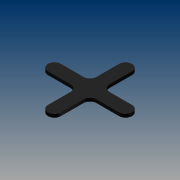
# Autodesk Inventor part: MotorBottom
Saved by Autodesk Inventor 2011 SP1 (Build 150282100, 282)
## iProperties
Created: 2011-07-19
Part Number: MotorBottom
Document SubType Name: Modeling
Designer: Nathan
Density: 1 g/cm^3
Author: Nathan
Autodesk Inventor part; units mm, degrees
ref_plane "YZ Plane" through (0, 0, 0) normal (1, 0, 0) x (0, 1, 0)
ref_plane "XZ Plane" through (0, 0, 0) normal (0, 1, 0) x (-1, 0, 0)
ref_plane "XY Plane" through (0, 0, 0) normal (0, 0, 1) x (1, 0, 0)
sketch "Sketch3" plane through (0, 0, 0) normal (0, 1, 0) x (-1, 0, 0)
  line L0 (-3.175, 3.175) -> (-3.175, 20.6375)
  line L1 (-3.175, 20.6375) -> (3.175, 20.6375)
  line L2 (3.175, 20.6375) -> (3.175, 3.175)
  line L3 (3.175, 3.175) -> (20.6375, 3.175)
  line L4 (20.6375, 3.175) -> (20.6375, -3.175)
  line L5 (20.6375, -3.175) -> (3.175, -3.175)
  line L6 (3.175, -3.175) -> (3.175, -20.6375)
  line L7 (3.175, -20.6375) -> (-3.175, -20.6375)
  line L8 (-3.175, -20.6375) -> (-3.175, -3.175)
  line L9 (-3.175, -3.175) -> (-20.6375, -3.175)
  line L10 (-20.6375, -3.175) -> (-20.6375, 3.175)
  line L11 (-20.6375, 3.175) -> (-3.175, 3.175)
  line L12 (0, 0) -> (2.5051, 0)
  line L13 (0, 0) -> (0, 2.7764)
  line L14 (0, 0) -> (2.5118, 2.5118)
  dimension "d17" = 45
  dimension "d18" = 6.35
  dimension "d19" = 20.6375
  dimension "d20" = 20.6375
  constraints: 30 end point, 9 parallel, 5 collinear, 2 horizontal, 2 perpendicular, 2 vertical, 1 point on line, 4 other
  measures "d17" angle of L14 L12
  measures "d18" distance of L0.end L1.end
  measures "d19" distance between parallel lines of L13 L4
  measures "d20" distance between parallel lines of L12 L1
extrude "Extrusion1" add sketch "Sketch3" along normal blind 1.5875
fillet "Fillet1" radius 3.175 1 edges at (-3.175, 0.7937, 20.6375)
fillet "Fillet2" radius 3.175 1 edges at (3.175, 0.7937, 20.6375)
fillet "Fillet3" radius 3.175 1 edges at (-20.6375, 0.7937, 3.175)
fillet "Fillet4" radius 3.175 1 edges at (-20.6375, 0.7937, -3.175)
fillet "Fillet5" radius 3.175 1 edges at (-3.175, 0.7937, -20.6375)
fillet "Fillet6" radius 3.175 1 edges at (3.175, 0.7937, -20.6375)
fillet "Fillet7" radius 3.175 1 edges at (20.6375, 0.7937, 3.175)
fillet "Fillet8" radius 3.175 1 edges at (20.6375, 0.7937, -3.175)
fillet "Fillet9" radius 3.175 1 edges at (3.175, 0.7937, 3.175)
fillet "Fillet10" radius 3.175 1 edges at (-3.175, 0.7937, 3.175)
fillet "Fillet11" radius 3.175 1 edges at (-3.175, 0.7937, -3.175)
fillet "Fillet12" radius 3.175 1 edges at (3.175, 0.7937, -3.175)
equation "\"d19\" = d20"
body "Solid2"
